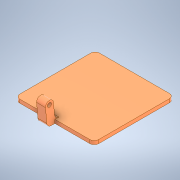
# Autodesk Inventor part: Tapas
Saved by Autodesk Inventor 2020.3 (Build 243373000, 373)
## iProperties
Created: 2020-08-31
Part Number: Tapas
Material: ABS Plastic
Document SubType Name: Modeling
Designer: juanp
Density: 1.06 g/cm^3
Appearance: Smooth - White
Author: juanp
Autodesk Inventor part; units mm, degrees
ref_plane "YZ Plane" through (0, 0, 0) normal (1, 0, 0) x (0, 1, 0)
ref_plane "XZ Plane" through (0, 0, 0) normal (0, 1, 0) x (-1, 0, 0)
ref_plane "XY Plane" through (0, 0, 0) normal (0, 0, 1) x (1, 0, 0)
sketch "Sketch1" plane through (0, 0, 0) normal (0, 1, 0) x (-1, 0, 0)
  line L0 (0, 0) -> (89.023, 0)
  line L1 (89.023, 0) -> (89.023, -90)
  line L2 (89.023, -90) -> (0, -90)
  line L3 (0, -90) -> (0, 0)
  dimension "d0" = 89.023
  dimension "d1" = 90
  constraints: 8 end point, 2 parallel, 1 horizontal, 1 perpendicular
  measures "d0" distance of L1.end L2.end
  measures "d1" distance of L0.end L1.end
extrude "Extrusion1" add sketch "Sketch1" along normal blind 4
ref_plane "Work Plane1" through (-44.5115, 0, 0) normal (1, 0, 0) x (0, 0, -1)
ref_plane "Work Plane2" through (-44.5115, 0, -90) normal (-1, 0, 0) x (0, 0, 1)
sketch "Sketch5" plane through (-44.5115, 0, -90) normal (-1, 0, 0) x (0, 0, 1)
  line L0 (90, 0) -> (90, 4) construction
  line L1 (90, 4) -> (96.1, 4) construction
  line L2 (96.1, 4) -> (96.1, 21.2) construction
  line L3 (96.1, 21.2) -> (90, 21.2) construction
  line L4 (90, 21.2) -> (90, 4) construction
  circle A0 centre (96.1, 21.2) radius 4.5
  line L5 (90, 0) -> (0, 0) projected
  line L6 (0, 0) -> (0, 4) projected
  line L7 (90, 4) -> (0, 4) projected
  line L8 (90, 0) -> (90, 4) projected
  line L9 (91.6189, 21.6119) -> (90.4175, 8.5423)
  line L10 (99.0878, 4.5423) -> (100.5811, 20.7881)
  line L11 (90, 0) -> (90, 4) projected
  line L12 (90, 0) -> (94.1088, 0)
  line L13 (85.4385, 4) -> (75.881, 4)
  line L14 (90, 4) -> (0, 4) projected
  arc A1 (85.4385, 4) -> (90.4175, 8.5423) centre (85.4385, 9) ccw
  arc A2 (94.1088, 0) -> (99.0878, 4.5423) centre (94.1088, 5) ccw
  point P0 (92.3607, 23.7035)
  dimension "d14" = 6.1
  dimension "d15" = 17.2
  dimension "d16" = 9
  dimension "d29" = 5
  constraints: 16 end point, 7 point on circle, 6 tangent, 3 centre point, 3 parallel, 3 point on line, 2 horizontal, 1 coincident, 1 equal radius, 1 perpendicular
  measures "d14" distance of L3.end L2.end
  measures "d15" distance of L2.end L1.end
  measures "d16" diameter of A0
  measures "d29" radius of A1
extrude "Extrusion4" add sketch "Sketch5" along normal blind 10 contours A0 | A0 L10 A2 L12 L8 L7 A1 L9
sketch "Sketch6" plane through (-44.5115, 0, -90) normal (1, 0, 0) x (0, 0, -1)
  arc A0 (-91.6189, 21.6119) -> (-100.5811, 20.7881) centre (-96.1, 21.2) ccw projected
  circle A1 centre (-96.1, 21.2) radius 2.3
  point P0 (-90, 0)
  point P1 (-99.8393, 18.6965)
  point P2 (-92.3607, 23.7035)
  dimension "d19" = 4.6
  constraints: 1 centre point, 1 coincident
  measures "d19" diameter of A1
extrude "Extrusion5" cut sketch "Sketch6" against normal blind 3.1
sketch "Sketch7" plane through (-54.5115, 0, -90) normal (-1, 0, 0) x (0, 0, 1)
  arc A0 (100.5811, 20.7881) -> (91.6189, 21.6119) centre (96.1, 21.2) ccw projected
  circle A1 centre (96.1, 21.2) radius 2.3
  point P0 (90, 0)
  point P1 (99.8393, 18.6965)
  point P2 (92.3607, 23.7035)
  dimension "d22" = 4.6
  constraints: 1 centre point, 1 coincident
  measures "d22" diameter of A1
extrude "Extrusion6" cut sketch "Sketch7" against normal blind 3.1
sketch "Sketch8" plane through (-51.4115, 21.2, 6.1) normal (-1, 0, 0) x (0, 0, 1)
  circle A0 centre (0, 0) radius 2.3 projected
  circle A1 centre (0, 0) radius 1
  point P0 (-6.1, -21.2)
  dimension "d25" = 2
  constraints: 1 centre point, 1 coincident
  measures "d25" diameter of A1
extrude "Extrusion7" cut sketch "Sketch8" against normal through all contours A1
fillet "Fillet2" radius 5 4 edges at (-89.023, 2, 0) (0, 2, 0) (0, 2, -90) (-89.023, 2, -90)
body "Solid1"
